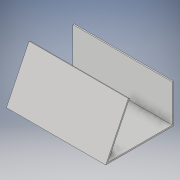
# Autodesk Inventor part: KartBuildArea
Saved by Autodesk Inventor 2018 (Build 220112000, 112)
## iProperties
Created: 2018-11-12
Part Number: KartBuildArea
Material: Generic
Document SubType Name: Modeling
Designer: tbrow
Density: 1 g/cm^3
Appearance: Default
Author: tbrow
Autodesk Inventor part; units mm, degrees
ref_plane "YZ Plane" through (0, 0, 0) normal (1, 0, 0) x (0, 1, 0)
ref_plane "XZ Plane" through (0, 0, 0) normal (0, 1, 0) x (-1, 0, 0)
ref_plane "XY Plane" through (0, 0, 0) normal (0, 0, 1) x (1, 0, 0)
sketch "Sketch1" plane through (0, 0, 0) normal (1, 0, 0) x (0, 1, 0)
  line L0 (0, 0) -> (-2.54, 0) construction
  line L1 (-2.54, 0) -> (-2.54, -127)
  line L2 (-2.54, -127) -> (0, -127) construction
  line L3 (0, -127) -> (0, 0)
  line L4 (0, 0) -> (87.664, -42.7566)
  line L5 (87.664, -42.7566) -> (88.7775, -40.4737)
  line L6 (88.7775, -40.4737) -> (-2.54, 4.0648)
  line L7 (-2.54, 4.0648) -> (-2.54, 0)
  line L8 (-2.54, -127) -> (73.66, -127) construction
  line L9 (73.66, -127) -> (73.66, -129.54)
  line L10 (73.66, -129.54) -> (-2.54, -129.54)
  line L11 (-2.54, -129.54) -> (-2.54, -127)
  line L12 (73.66, -127) -> (0, -127)
  dimension "d0" = 127
  dimension "d1" = 2.54
  dimension "d2" = 2.54
  dimension "d3" = 101.6
  dimension "d4" = 64
  dimension "d5" = 76.2
  dimension "d6" = 2.54
  constraints: 26 end point, 4 parallel, 4 perpendicular, 2 horizontal, 1 collinear, 1 vertical
  measures "d0" distance of L0.end L1.end
  measures "d1" distance of L1.end L2.end
  measures "d2" distance between parallel lines of L4 L6
  measures "d3" distance of L5.end L6.end
  measures "d4" angle of L3 L4
  measures "d5" distance of L9.end L10.end
  measures "d6" distance of L8.end L9.end
extrude "Extrusion1" add sketch "Sketch1" along normal blind 195.58
body "Solid1"
